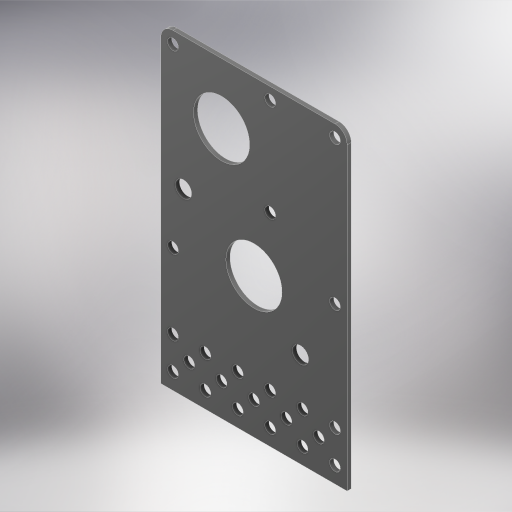
# Autodesk Inventor part: POM 1
Saved by Autodesk Inventor 2024 (Build 280153000, 153)
## iProperties
Created: 2023-09-01
Part Number: POM 1
Material: Acetal Resin, Black
Document SubType Name: Modeling
Designer: aaron
Density: 1.425 g/cm^3
Appearance: Smooth - Black
Author: aaron
Autodesk Inventor part; units mm, degrees
ref_plane "YZ Plane" through (0, 0, 0) normal (1, 0, 0) x (0, 1, 0)
ref_plane "XZ Plane" through (0, 0, 0) normal (0, 1, 0) x (-1, 0, 0)
ref_plane "XY Plane" through (0, 0, 0) normal (0, 0, 1) x (1, 0, 0)
sketch "Sketch1" plane through (0, 0, 0) normal (0, 0, 1) x (1, 0, 0)
  line L0 (57.15, -58.7375) -> (-57.15, -58.7375)
  line L1 (-57.15, -58.7375) -> (-57.15, 58.7375)
  line L2 (-57.15, 58.7375) -> (57.15, 58.7375)
  line L3 (57.15, 58.7375) -> (57.15, -58.7375)
  line L4 (57.15, -58.7375) -> (-57.15, 58.7375) construction
  line L5 (-57.15, -58.7375) -> (57.15, 58.7375) construction
  line L6 (-57.15, 58.7375) -> (-19.05, 58.7375)
  line L7 (-19.05, 58.7375) -> (-19.05, 20.6375)
  line L8 (-19.05, 20.6375) -> (-57.15, 20.6375)
  line L9 (-57.15, 20.6375) -> (-57.15, 58.7375)
  circle A0 centre (-38.1, 39.6875) radius 19.05
  circle A1 centre (-57.15, 58.7375) radius 4.7625
  circle A2 centre (57.15, 58.7375) radius 4.7625
  line L10 (-57.15, -58.7375) -> (-61.9125, -58.7375)
  line L11 (-61.9125, -58.7375) -> (-61.9125, 58.7375)
  line L12 (57.15, -58.7375) -> (61.9125, -58.7375)
  line L13 (61.9125, -58.7375) -> (61.9125, 58.7375)
  line L14 (57.15, 63.5) -> (-57.15, 63.5)
  circle A3 centre (-38.1, 39.6875) radius 10.9855
  circle A4 centre (-57.15, 58.7375) radius 2.1082
  circle A5 centre (57.15, 58.7375) radius 2.1082
  point P0 (0, 0)
  dimension "d0" = 114.3
  dimension "d1" = 117.475
  dimension "d2" = 38.1
  dimension "d3" = 38.1
  dimension "d4" = 9.525
  dimension "d5" = 9.525
  dimension "d6" = 4.7625
  dimension "d7" = 4.7625
  dimension "d8" = 21.971
  dimension "d9" = 4.2164
  dimension "d10" = 4.2164
  constraints: 30 end point, 6 centre point, 5 coincident, 4 horizontal, 4 parallel, 4 perpendicular, 4 point on circle, 3 tangent, 2 midpoint
  measures "d0" distance of L1.end L2.end
  measures "d1" distance of L0.end L1.end
  measures "d2" distance of L7.end L8.end
  measures "d3" distance of L6.end L7.end
  measures "d4" diameter of A1
  measures "d5" diameter of A2
  measures "d6" distance of L0.end L10.end
  measures "d7" distance of L0.start L12.end
  measures "d8" diameter of A3
  measures "d9" diameter of A4
  measures "d10" diameter of A5
extrude "Extrusion1" add sketch "Sketch1" along normal blind 1.5875 contours L0 L1 L8 L7 L2 A2 L3 | L3 A2 L13 L12 | L10 L11 A1 L1 | A2 L2 A5 L3 | L3 A5 L2 A2 | L1 A0 L8 | L2 A1 L14 A2 | L1 A1 L2 A0 | A0 | A0 L7 L8 | A1 L2 A4 L1 | L7 A0 L2 | L1 A4 L2 A1
sketch "Sketch2" plane through (0, 0, 1.5875) normal (0, 0, 1) x (1, 0, 0)
  circle A0 centre (-38.1, 39.6875) radius 10.9855 projected
  line L0 (-38.1, 39.6875) -> (61.9125, 39.6875)
  line L1 (61.9125, -58.7375) -> (61.9125, 58.7375) projected
  circle A1 centre (-38.1, 39.6875) radius 6.35
  circle A2 centre (-12.7, 39.6875) radius 19.05
  circle A3 centre (38.1, 39.6875) radius 31.75
  circle A4 centre (-12.7, 39.6875) radius 10.9855
  circle A5 centre (38.1, 39.6875) radius 10.9855
  line L2 (-61.9125, 58.7375) -> (-61.9125, -58.7375) projected
  line L3 (-61.9125, -3.9688) -> (61.9125, -3.9688)
  line L4 (-38.1, 39.6875) -> (-12.7, 39.6875)
  line L5 (-25.4, 39.6875) -> (-25.4, -3.9688)
  circle A6 centre (-25.4, -3.9688) radius 10.9855
  line L6 (57.15, 63.5) -> (-57.15, 63.5) projected
  line L7 (-61.9125, -58.7375) -> (61.9125, -58.7375) projected
  line L8 (0, -58.7375) -> (0, 63.5)
  circle A7 centre (0, -46.0375) radius 19.05
  circle A8 centre (0, -46.0375) radius 2.1082
  point P0 (0, 0)
  dimension "d13" = 12.7
  dimension "d14" = 38.1
  dimension "d15" = 63.5
  dimension "d16" = 21.971
  dimension "d17" = 21.971
  dimension "d18" = 43.6562
  dimension "d19" = 21.971
  dimension "d20" = 25.4
  dimension "d21" = 38.1
  dimension "d22" = 12.7
  dimension "d23" = 4.2164
  constraints: 10 end point, 8 centre point, 7 point on line, 5 coincident, 3 midpoint, 2 perpendicular, 2 tangent, 1 collinear, 1 horizontal, 1 vertical
  measures "d13" diameter of A1
  measures "d14" diameter of A2
  measures "d15" diameter of A3
  measures "d16" diameter of A4
  measures "d17" diameter of A5
  measures "d18" distance between parallel lines of L3 L0
  measures "d19" diameter of A6
  measures "d20" distance between parallel lines of L5 L8
  measures "d21" diameter of A7
  measures "d22" distance from line of L7 A7.centre
  measures "d23" diameter of A8
extrude "Extrusion2" cut sketch "Sketch2" against normal blind 1.5875 contours A4 L0 | L0 A4 | A6 L3 L5 | L5 L3 A6 | A5 L0 | L0 A5 | L3 A6 | A8 L8 | L8 A8
sketch "Sketch3" plane through (0, 0, 1.5875) normal (0, 0, 1) x (1, 0, 0)
  circle A0 centre (-25.4, -3.9688) radius 10.9855 projected
  circle A1 centre (-38.1, 39.6875) radius 10.9855 projected
  circle A2 centre (0, -46.0375) radius 2.1082 projected
  circle A3 centre (0, -46.0375) radius 19.05
  circle A4 centre (-25.4, -3.9688) radius 19.05
  circle A5 centre (-38.1, 39.6875) radius 19.05
  circle A6 centre (-53.0324, 11.6681) radius 12.7
  circle A7 centre (-7.1902, -21.6764) radius 6.35
  circle A8 centre (-53.0324, 11.6681) radius 3.175
  circle A9 centre (-7.1902, -21.6764) radius 3.175
  point P0 (0, 0)
  dimension "d26" = 38.1
  dimension "d27" = 38.1
  dimension "d28" = 38.1
  dimension "d29" = 25.4
  dimension "d30" = 12.7
  dimension "d31" = 6.35
  dimension "d32" = 6.35
  constraints: 7 centre point, 5 coincident, 4 tangent
  measures "d26" diameter of A3
  measures "d27" diameter of A4
  measures "d28" diameter of A5
  measures "d29" diameter of A6
  measures "d30" diameter of A7
  measures "d31" diameter of A8
  measures "d32" diameter of A9
extrude "Extrusion3" cut sketch "Sketch3" against normal blind 25.4 contours A8 | A9
sketch "Sketch4" plane through (0, 0, 1.5875) normal (0, 0, 1) x (1, 0, 0)
  circle A0 centre (0, -46.0375) radius 2.1082 projected
  line L0 (0, -46.0375) -> (-6.35, -46.0375)
  line L1 (-6.35, -46.0375) -> (-6.35, -39.6875)
  line L2 (-6.35, -39.6875) -> (0, -39.6875)
  line L3 (0, -39.6875) -> (0, -46.0375)
  circle A1 centre (-6.35, -39.6875) radius 2.1082
  line L4 (-61.9125, -58.7375) -> (61.9125, -58.7375) projected
  line L5 (-61.9125, 58.7375) -> (-61.9125, -58.7375) projected
  circle A2 centre (6.35, -39.6875) radius 2.1082
  circle A3 centre (19.05, -39.6875) radius 2.1082
  circle A4 centre (31.75, -39.6875) radius 2.1082
  circle A5 centre (44.45, -39.6875) radius 2.1082
  circle A6 centre (57.15, -39.6875) radius 2.1082
  circle A7 centre (-6.35, -52.3875) radius 2.1082
  circle A8 centre (6.35, -52.3875) radius 2.1082
  circle A9 centre (19.05, -52.3875) radius 2.1082
  circle A10 centre (31.75, -52.3875) radius 2.1082
  circle A11 centre (44.45, -52.3875) radius 2.1082
  circle A12 centre (57.15, -52.3875) radius 2.1082
  circle A13 centre (-19.05, -39.6875) radius 2.1082
  circle A14 centre (-31.75, -39.6875) radius 2.1082
  circle A15 centre (-44.45, -39.6875) radius 2.1082
  circle A16 centre (-57.15, -39.6875) radius 2.1082
  circle A17 centre (-6.35, -52.3875) radius 2.1082
  circle A18 centre (-19.05, -52.3875) radius 2.1082
  circle A19 centre (-31.75, -52.3875) radius 2.1082
  circle A20 centre (-44.45, -52.3875) radius 2.1082
  circle A21 centre (-57.15, -52.3875) radius 2.1082
  point P0 (0, 0)
  dimension "d35" = 6.35
  dimension "d36" = 6.35
  dimension "d37" = 4.2164
  dimension "d40" = 12.7
  dimension "d43" = 12.7
  dimension "d48" = 12.7
  dimension "d51" = 12.7
  constraints: 21 centre point, 8 end point, 3 horizontal, 2 parallel, 2 vertical, 1 coincident, 1 perpendicular, 40 other
  measures "d35" distance of L1.end L2.end
  measures "d36" distance of L0.end L1.end
  measures "d37" diameter of A1
  measures "d40" distance of A1.centre A2.centre
  measures "d43" distance of A1.centre A7.centre
  measures "d48" distance of A1.centre A13.centre
  measures "d51" distance of A1.centre A17.centre
extrude "Extrusion4" cut sketch "Sketch4" against normal blind 25.4 contours A1 L1 L2 | L2 L1 A1 | A2 | A3 | A4 | A5 | A6 | A7 | A8 | A9 | A10 | A11 | A12 | A13 | A14 | A15 | A16 | A18 | A19 | A20 | A21
sketch "Sketch7" plane through (0, 0, 1.5875) normal (0, 0, 1) x (1, 0, 0)
  circle A0 centre (-12.7, 39.6875) radius 10.9855 projected
  line L0 (12.7, 14.2875) -> (-38.1, 14.2875)
  line L1 (-38.1, 14.2875) -> (-38.1, 65.0875)
  line L2 (-38.1, 65.0875) -> (12.7, 65.0875)
  line L3 (12.7, 65.0875) -> (12.7, 14.2875)
  line L4 (12.7, 14.2875) -> (-38.1, 65.0875) construction
  line L5 (-38.1, 14.2875) -> (12.7, 65.0875) construction
  circle A1 centre (-38.1, 39.6875) radius 10.9855 projected
  circle A2 centre (-57.15, 58.7375) radius 2.1082 projected
  line L6 (-31.75, 20.6375) -> (6.35, 20.6375)
  line L7 (6.35, 20.6375) -> (6.35, 58.7375)
  line L8 (6.35, 58.7375) -> (-31.75, 58.7375)
  line L9 (-31.75, 58.7375) -> (-31.75, 20.6375)
  line L10 (-31.75, 20.6375) -> (6.35, 58.7375) construction
  line L11 (6.35, 20.6375) -> (-31.75, 58.7375) construction
  circle A3 centre (6.35, 58.7375) radius 2.1082
  circle A4 centre (6.35, 58.7375) radius 4.7625
  line L12 (11.1125, 58.7375) -> (11.1125, -58.7375)
  line L13 (-61.9125, -58.7375) -> (61.9125, -58.7375) projected
  line L14 (-61.9125, -58.7375) -> (61.9125, -58.7375) projected
  circle A5 centre (-25.4, -3.9688) radius 10.9855 projected
  circle A6 centre (-25.4, -3.9688) radius 2.1082
  line L15 (-25.4, -3.9688) -> (-31.75, -3.9688)
  line L16 (-31.75, -3.9688) -> (-31.75, 2.3812)
  line L17 (-31.75, 2.3812) -> (-25.4, 2.3812)
  line L18 (-25.4, 2.3812) -> (-25.4, -3.9688)
  circle A7 centre (-31.75, 2.3812) radius 2.1082
  circle A8 centre (-38.1, -3.9688) radius 2.1082
  circle A9 centre (-50.8, -3.9688) radius 2.1082
  circle A10 centre (-12.7, -3.9688) radius 2.1082
  circle A11 centre (-25.4, -3.9688) radius 2.1082
  circle A12 centre (-38.1, -3.9688) radius 2.1082
  circle A13 centre (0, -3.9688) radius 2.1082
  circle A14 centre (-12.7, -3.9688) radius 2.1082
  circle A15 centre (-25.4, -3.9688) radius 2.1082
  circle A16 centre (-44.45, 2.3812) radius 2.1082
  circle A17 centre (-57.15, 2.3812) radius 2.1082
  circle A18 centre (-31.75, -10.3188) radius 2.1082
  circle A19 centre (-44.45, -10.3188) radius 2.1082
  circle A20 centre (-57.15, -10.3188) radius 2.1082
  circle A21 centre (-19.05, 2.3812) radius 2.1082
  circle A22 centre (-6.35, 2.3812) radius 2.1082
  circle A23 centre (6.35, 2.3812) radius 2.1082
  circle A24 centre (-31.75, -10.3188) radius 2.1082
  circle A25 centre (-19.05, -10.3188) radius 2.1082
  circle A26 centre (-6.35, -10.3188) radius 2.1082
  circle A27 centre (6.35, -10.3188) radius 2.1082
  line L19 (57.15, 63.5) -> (-57.15, 63.5) projected
  line L20 (61.9125, -58.7375) -> (61.9125, 58.7375) projected
  line L21 (11.1125, 58.7375) -> (61.9125, 58.7375)
  line L22 (61.9125, 58.7375) -> (61.9125, -58.7375)
  line L23 (61.9125, -58.7375) -> (11.1125, -58.7375)
  line L24 (11.1125, -58.7375) -> (11.1125, 58.7375)
  line L25 (61.9125, -58.7375) -> (61.9125, 58.7375) projected
  arc A28 (61.9125, 58.7375) -> (57.15, 63.5) centre (57.15, 58.7375) ccw projected
  point P0 (0, 0)
  point P1 (6.35, 63.5)
  dimension "d71" = 9.525
  dimension "d66" = 50.8
  dimension "d67" = 50.8
  dimension "d68" = 38.1
  dimension "d69" = 38.1
  dimension "d70" = 4.2164
  dimension "d72" = 4.2164
  dimension "d73" = 6.35
  dimension "d74" = 6.35
  dimension "d75" = 4.2164
  dimension "d78" = 12.7
  dimension "d81" = 12.7
  dimension "d86" = 12.7
  dimension "d89" = 12.7
  dimension "d94" = 12.7
  dimension "d97" = 12.7
  constraints: 42 end point, 23 centre point, 8 horizontal, 8 parallel, 5 perpendicular, 4 coincident, 4 midpoint, 4 vertical, 1 point on line, 43 other
  measures "d66" distance of L1.end L2.end
  measures "d67" distance of L0.end L1.end
  measures "d68" distance of L8.end L7.end
  measures "d69" distance of L7.end L6.end
  measures "d70" diameter of A3
  measures "d72" diameter of A6
  measures "d73" distance of L16.end L17.end
  measures "d74" distance of L15.end L16.end
  measures "d75" diameter of A7
  measures "d78" distance of L15.start A8.centre
  measures "d81" distance of L15.start A10.centre
  measures "d86" distance of A7.centre A16.centre
  measures "d89" distance of A7.centre A18.centre
  measures "d94" distance of A7.centre A21.centre
  measures "d97" distance of A7.centre A24.centre
extrude "Extrusion6" cut sketch "Sketch7" against normal blind 25.4 contours L3 L21 L20 L13 L12 L0 | L0 L12 L21 L3 | L21 A4 L19 L3 | L3 L19 A28 L21 | A3 L8 L7 | L7 L8 A3
sketch "Sketch9" plane through (0, 0, 1.5875) normal (0, 0, 1) x (1, 0, 0)
  circle A0 centre (0, -46.0375) radius 2.1082 projected
  circle A1 centre (0, -46.0375) radius 2.1082
  line L0 (-61.9125, -58.7375) -> (11.1125, -58.7375) projected
  circle A2 centre (-12.7, -46.0375) radius 2.1082
  circle A3 centre (-25.4, -46.0375) radius 2.1082
  circle A4 centre (-38.1, -46.0375) radius 2.1082
  circle A5 centre (-50.8, -46.0375) radius 2.1082
  point P0 (0, 0)
  dimension "d117" = 12.7
  constraints: 5 centre point, 1 coincident, 1 concentric, 1 horizontal, 8 other
  measures "d117" distance of A1.centre A2.centre
extrude "Extrusion8" cut sketch "Sketch9" against normal blind 25.4
sketch "Sketch10" plane through (0, 0, 1.5875) normal (0, 0, 1) x (1, 0, 0)
  circle A0 centre (-12.7, 39.6875) radius 10.9855 projected
  point P0 (0, 0)
extrude "Extrusion9" add sketch "Sketch10" against normal blind 1.5875
sketch "Sketch11" plane through (0, 0, 1.5875) normal (0, 0, 1) x (1, 0, 0)
  circle A0 centre (-25.4, -3.9688) radius 10.9855 projected
  line L0 (-25.4, -3.9688) -> (-57.15, -3.9688)
  line L1 (-57.15, -3.9688) -> (-57.15, -10.3188)
  line L2 (-57.15, -10.3188) -> (-25.4, -10.3188)
  line L3 (-25.4, -10.3188) -> (-25.4, -3.9688)
  circle A1 centre (-57.15, -10.3188) radius 2.1082
  point P0 (0, 0)
  dimension "d126" = 31.75
  dimension "d127" = 6.35
  dimension "d128" = 4.2164
  constraints: 8 end point, 2 parallel, 1 centre point, 1 coincident, 1 horizontal, 1 perpendicular
  measures "d126" distance of L2.end L1.end
  measures "d127" distance of L1.end L0.end
  measures "d128" diameter of A1
extrude "Extrusion10" cut sketch "Sketch11" against normal blind 1.5875 contours A1 L1 L2 | L2 L1 A1
sketch "Sketch12" plane through (0, 0, 1.5875) normal (0, 0, 1) x (1, 0, 0)
  circle A0 centre (-38.1, 39.6875) radius 10.9855 projected
  line L0 (-57.15, 58.7375) -> (-19.05, 58.7375)
  line L1 (-19.05, 58.7375) -> (-19.05, 20.6375)
  line L2 (-19.05, 20.6375) -> (-57.15, 20.6375)
  line L3 (-57.15, 20.6375) -> (-57.15, 58.7375)
  line L4 (-57.15, 58.7375) -> (-19.05, 20.6375) construction
  line L5 (-19.05, 58.7375) -> (-57.15, 20.6375) construction
  circle A1 centre (-19.05, 58.7375) radius 2.1082
  circle A2 centre (-19.05, 20.6375) radius 2.1082
  point P0 (0, 0)
  dimension "d131" = 38.1
  dimension "d132" = 38.1
  dimension "d133" = 4.2164
  dimension "d134" = 4.2164
  constraints: 12 end point, 2 centre point, 2 coincident, 2 midpoint, 2 parallel, 1 horizontal, 1 perpendicular
  measures "d131" distance of L1.end L2.end
  measures "d132" distance of L0.end L1.end
  measures "d133" diameter of A1
  measures "d134" diameter of A2
extrude "Extrusion11" cut sketch "Sketch12" against normal blind 1.5875 contours A1 L1 L0 | L0 L1 A1 | A2 L1 L2 | L2 L1 A2
sketch "Sketch13" plane through (0, 0, 1.5875) normal (0, 0, 1) x (1, 0, 0)
  circle A0 centre (-25.4, -3.9688) radius 10.9855 projected
  line L0 (-25.4, -3.9688) -> (6.35, -3.9688)
  line L1 (6.35, -3.9688) -> (6.35, 2.3812)
  line L2 (6.35, 2.3812) -> (-25.4, 2.3812)
  line L3 (-25.4, 2.3812) -> (-25.4, -3.9688)
  circle A1 centre (6.35, 2.3812) radius 2.1082
  point P0 (0, 0)
  dimension "d137" = 31.75
  dimension "d138" = 6.35
  dimension "d139" = 4.2164
  constraints: 8 end point, 2 parallel, 1 centre point, 1 coincident, 1 horizontal, 1 perpendicular
  measures "d137" distance of L2.end L1.end
  measures "d138" distance of L1.end L0.end
  measures "d139" diameter of A1
extrude "Extrusion12" cut sketch "Sketch13" against normal blind 1.5875 contours A1 L1 L2 | L2 L1 A1
body "Solid1"
